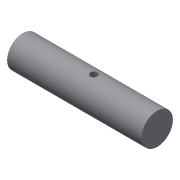
# Autodesk Inventor part: shaft
Saved by Autodesk Inventor 2022 (Build 260148000, 148)
## iProperties
Created: 2005-10-24
Part Number: shaft
Document SubType Name: Modeling
Designer: dchu
Density: 1 g/cm^3
Material: Generic
Appearance: Default
Author: dchu
Autodesk Inventor part; units mm, degrees
ref_plane "YZ Plane" through (0, 0, 0) normal (1, 0, 0) x (0, 1, 0)
ref_plane "XZ Plane" through (0, 0, 0) normal (0, 1, 0) x (-1, 0, 0)
sketch "Sketch1" plane through (0, 0, 0) normal (1, 0, 0) x (0, 1, 0)
  circle A0 centre (0, 0) radius 17.5
  dimension "d0" = 35
  constraints: 1 centre point
  measures "d0" diameter of A0
extrude "Extrusion1" add sketch "Sketch1" along normal mid plane 150
ref_plane "Work Plane1" through (75, 0, -17.5) normal (0, 0, 1) x (-1, 0, 0)
sketch "Sketch2" plane through (75, 0, -17.5) normal (0, 0, 1) x (-1, 0, 0)
  line L0 (-45, 0) -> (165, 0) projected
  line L1 (150, 17.5) -> (0, 17.5) projected
  point P0 (70.5604, 0)
  constraints: 1 point on line
hole "Hole1" at (4.4396, 0, -17.5) direction (0, 0, 1) diameter 8 end through all
body "Solid1"
